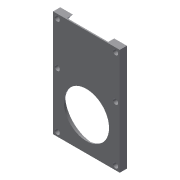
# Autodesk Inventor part: 200_Gearbox
Saved by Autodesk Inventor 2019 (Build 230136000, 136)
## iProperties
Created: 2019-07-08
Part Number: 200_Gearbox
Material: Generic
Document SubType Name: Modeling
Designer: diederichbenedict
Density: 1 g/cm^3
Appearance: Default
Author: diederichbenedict
Autodesk Inventor part; units mm, degrees
ref_plane "YZ Plane" through (0, 0, 0) normal (1, 0, 0) x (0, 1, 0)
ref_plane "XZ Plane" through (0, 0, 0) normal (0, 1, 0) x (-1, 0, 0)
ref_plane "XY Plane" through (0, 0, 0) normal (0, 0, 1) x (1, 0, 0)
sketch "Sketch1" plane through (0, 0, 0) normal (0, 0, 1) x (1, 0, 0)
  circle A0 centre (7.7782, 0) radius 0.9 construction
  circle A1 centre (-7.7782, 0) radius 0.9 construction
  circle A2 centre (0, -7.7782) radius 0.9 construction
  circle A3 centre (0, 7.7782) radius 0.9 construction
  arc A4 (0, 10) -> (-2.698, 9.6292) centre (0, 0) ccw construction
  arc A5 (-2.698, 9.6292) -> (-5.1958, 8.5442) centre (0, 0) ccw construction
  arc A6 (-5.1958, 8.5442) -> (-7.3084, 6.8255) centre (0, 0) ccw construction
  arc A7 (-7.3084, 6.8255) -> (-8.8789, 4.6007) centre (0, 0) ccw construction
  arc A8 (-8.8789, 4.6007) -> (-9.7908, 2.0346) centre (0, 0) ccw construction
  arc A9 (-9.7908, 2.0346) -> (-9.9767, -0.6824) centre (0, 0) ccw construction
  arc A10 (-9.9767, -0.6824) -> (-9.4226, -3.3488) centre (0, 0) ccw construction
  arc A11 (-9.4226, -3.3488) -> (-8.1697, -5.7668) centre (0, 0) ccw construction
  arc A12 (-8.1697, -5.7668) -> (-6.3109, -7.7571) centre (0, 0) ccw construction
  arc A13 (-6.3109, -7.7571) -> (-3.984, -9.1721) centre (0, 0) ccw construction
  arc A14 (-3.984, -9.1721) -> (-1.3617, -9.9069) centre (0, 0) ccw construction
  arc A15 (-1.3617, -9.9069) -> (1.3617, -9.9069) centre (0, 0) ccw construction
  arc A16 (1.3617, -9.9069) -> (3.984, -9.1721) centre (0, 0) ccw construction
  arc A17 (3.984, -9.1721) -> (6.3109, -7.7571) centre (0, 0) ccw construction
  arc A18 (6.3109, -7.7571) -> (8.1697, -5.7668) centre (0, 0) ccw construction
  arc A19 (8.1697, -5.7668) -> (9.4226, -3.3488) centre (0, 0) ccw construction
  arc A20 (9.4226, -3.3488) -> (9.9767, -0.6824) centre (0, 0) ccw construction
  arc A21 (9.9767, -0.6824) -> (9.7908, 2.0346) centre (0, 0) ccw construction
  arc A22 (9.7908, 2.0346) -> (8.8789, 4.6007) centre (0, 0) ccw construction
  arc A23 (8.8789, 4.6007) -> (7.3084, 6.8255) centre (0, 0) ccw construction
  arc A24 (7.3084, 6.8255) -> (5.1958, 8.5442) centre (0, 0) ccw construction
  arc A25 (5.1958, 8.5442) -> (2.698, 9.6292) centre (0, 0) ccw construction
  arc A26 (2.698, 9.6292) -> (0, 10) centre (0, 0) ccw construction
  arc A27 (-7.3084, 9.5178) -> (7.3084, 9.5178) centre (0, 0) ccw
  arc A28 (8.2415, 16.5957) -> (9.4944, 19.0137) centre (0.0718, 22.3625) ccw construction
  line L0 (14, -14) -> (-14, -14)
  line L1 (-14, -14) -> (-14, 30.6843)
  line L2 (14, 30.6843) -> (14, -14)
  line L3 (7.3084, 12.4534) -> (7.3084, 9.5178)
  line L4 (-7.3084, 12.4534) -> (-7.3084, 9.5178)
  arc A29 (7.3084, 12.4534) -> (8.6716, 30.6843) centre (0, 22.1663) ccw
  arc A30 (-8.6716, 30.6843) -> (-7.3084, 12.4534) centre (0, 22.1663) ccw
  line L5 (-14, 30.6843) -> (-8.6716, 30.6843)
  line L6 (8.6716, 30.6843) -> (14, 30.6843)
  line L7 (-3.5, -3.5) -> (-3.5, 3.5) projected
  line L8 (-3.5, 3.5) -> (3.5, 3.5) projected
  line L9 (3.5, 3.5) -> (3.5, -3.5) projected
  line L10 (3.5, -3.5) -> (-3.5, -3.5) projected
  point P0 (10.0485, 21.6801)
  dimension "d0" = 24
  dimension "d1" = 14
  dimension "d2" = 14
  dimension "d3" = 14
  constraints: 14 end point, 6 point on circle, 3 centre point, 3 parallel, 1 coincident, 1 horizontal, 1 perpendicular, 1 other
  measures "d0" diameter of A27
  measures "d1" distance from line of point (0, 0) L2
  measures "d2" distance from line of L1 point (0, 0)
  measures "d3" distance from line of L0 point (0, 0)
extrude "Extrusion1" add sketch "Sketch1" against normal blind 2.5 contours A27 L3 A29 L6 L2 L0 L1 L5 A30 L4
sketch "Sketch2" plane through (0, 0, 0) normal (0, 0, 1) x (1, 0, 0)
  line L0 (14, -14) -> (-14, -14) projected
  line L1 (14, 30.6843) -> (14, -14) projected
  line L2 (8.6716, 30.6843) -> (14, 30.6843) projected
  arc A0 (7.3084, 12.4534) -> (8.6716, 30.6843) centre (0, 22.1663) ccw projected
  line L3 (7.3084, 9.5178) -> (7.3084, 12.4534) projected
  arc A1 (-7.3084, 9.5178) -> (7.3084, 9.5178) centre (0, 0) ccw projected
  line L4 (-7.3084, 12.4534) -> (-7.3084, 9.5178) projected
  arc A2 (-8.6716, 30.6843) -> (-7.3084, 12.4534) centre (0, 22.1663) ccw projected
  line L5 (-14, 30.6843) -> (-8.6716, 30.6843) projected
  line L6 (-14, -14) -> (-14, 30.6843) projected
  circle A3 centre (0, 0) radius 8
  line L7 (-14, 30.6843) -> (-8.6716, 30.6843) projected
  line L8 (8.6716, 30.6843) -> (-8.6716, 30.6843)
  dimension "d6" = 16
  constraints: 2 end point, 1 centre point, 1 coincident, 1 collinear
  measures "d6" diameter of A3
extrude "Extrusion2" add sketch "Sketch2" along normal blind 0.5
sketch "Sketch3" plane through (0, 0, -2.5) normal (0, 0, -1) x (-1, 0, 0)
  line L0 (-14, -14) -> (14, -14) projected
  line L1 (14, -14) -> (14, 30.6843) projected
  line L2 (14, 30.6843) -> (8.6716, 30.6843) projected
  arc A0 (7.3084, 12.4534) -> (8.6716, 30.6843) centre (0, 22.1663) ccw projected
  line L3 (7.3084, 12.4534) -> (7.3084, 9.5178) projected
  arc A1 (-7.3084, 9.5178) -> (7.3084, 9.5178) centre (0, 0) ccw projected
  line L4 (-7.3084, 9.5178) -> (-7.3084, 12.4534) projected
  arc A2 (-8.6716, 30.6843) -> (-7.3084, 12.4534) centre (0, 22.1663) ccw projected
  line L5 (-8.6716, 30.6843) -> (-14, 30.6843) projected
  line L6 (-14, 30.6843) -> (-14, -14) projected
  line L7 (12.2447, 28.929) -> (12.2447, -12.2447) construction
  line L8 (12.2447, -12.2447) -> (-12.2447, -12.2447) construction
  line L9 (-12.2447, -12.2447) -> (-12.2447, 28.929) construction
  line L10 (-12.2447, 28.929) -> (-12.1562, 28.929) construction
  arc A3 (-12.1562, 28.929) -> (-9.0637, 11.6137) centre (0, 22.1663) ccw construction
  line L11 (-9.0637, 11.6137) -> (-9.0637, 10.3469) construction
  arc A4 (-9.0637, 10.3469) -> (9.0637, 10.3469) centre (0, 0) ccw construction
  line L12 (9.0637, 10.3469) -> (9.0637, 11.6137) construction
  arc A5 (9.0637, 11.6137) -> (12.1562, 28.929) centre (0, 22.1663) ccw construction
  line L13 (12.1562, 28.929) -> (12.2447, 28.929) construction
  point P0 (12.2447, 10.9803)
  point P1 (-12.2447, 10.9803)
  constraints: 14 end point, 6 point on circle, 3 centre point, 2 point on line, 9 other
hole "Hole1" at (-12.2447, 10.9803, -2.5) at (12.2447, 10.9803, -2.5) at (-12.2447, 28.929, -2.5) at (-12.2447, -12.2447, -2.5) at (12.2447, -12.2447, -2.5) at (12.2447, 28.929, -2.5) direction (0, 0, 1) diameter 2.15 depth 16 tip angle 118
body "Solid1"
